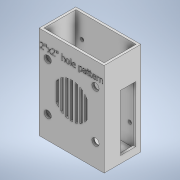
# Autodesk Inventor part: piCaseAttachesToTripodClamp
Saved by Autodesk Inventor 2022.1 (Build 261234020, 234B)
## iProperties
Created: 2021-02-07
Part Number: piCaseAttachesToTripodClamp
Material: Generic
Document SubType Name: Modeling
Designer: robst
Density: 1 g/cm^3
Appearance: Default
Author: robst
Autodesk Inventor part; units mm, degrees
ref_plane "YZ Plane" through (0, 0, 0) normal (1, 0, 0) x (0, 1, 0)
ref_plane "XZ Plane" through (0, 0, 0) normal (0, 1, 0) x (-1, 0, 0)
ref_plane "XY Plane" through (0, 0, 0) normal (0, 0, 1) x (1, 0, 0)
sketch "Sketch14" plane through (0, 0, 0) normal (0, 0, 1) x (1, 0, 0)
  line L0 (-34.54, -49.54) -> (34.54, -49.54)
  line L1 (34.54, -49.54) -> (34.54, 49.54)
  line L2 (34.54, 49.54) -> (-34.54, 49.54)
  line L3 (-34.54, 49.54) -> (-34.54, -49.54)
  line L4 (-34.54, -49.54) -> (34.54, 49.54) construction
  line L5 (34.54, -49.54) -> (-34.54, 49.54) construction
  point P0 (0, 0)
  dimension "d66" = 69.08
  dimension "d67" = 99.08
  constraints: 12 end point, 2 midpoint, 2 parallel, 1 horizontal, 1 perpendicular
  measures "d66" distance of L0.start L0.end
  measures "d67" distance of L2.end L0.start
extrude "Extrusion9" add sketch "Sketch14" against normal blind 2.54
sketch "Sketch15" plane through (0, 0, 0) normal (0, 0, 1) x (1, 0, 0)
  line L0 (-34.54, -49.54) -> (-34.54, 49.54) projected
  line L1 (34.54, 49.54) -> (34.54, -49.54) projected
  line L2 (-34.54, -49.54) -> (34.54, -49.54)
  line L3 (34.54, -49.54) -> (34.54, 49.54)
  line L4 (34.54, 49.54) -> (-34.54, 49.54)
  line L5 (-34.54, 49.54) -> (-34.54, -49.54)
  line L6 (-32, -47) -> (32, -47)
  line L7 (32, -47) -> (32, 47)
  line L8 (32, 47) -> (-32, 47)
  line L9 (-32, 47) -> (-32, -47)
  line L10 (-32, -47) -> (32, 47) construction
  line L11 (32, -47) -> (-32, 47) construction
  point P0 (0, 0)
  point P1 (34.54, -49.54)
  dimension "d70" = 64
  dimension "d71" = 94
  constraints: 20 end point, 4 parallel, 2 horizontal, 2 midpoint, 2 perpendicular
  measures "d70" distance of L6.start L6.end
  measures "d71" distance of L8.end L6.start
extrude "Extrusion10" add sketch "Sketch15" along normal blind 34
sketch "Sketch16" plane through (0, 0, 34) normal (0, 0, 1) x (1, 0, 0)
  line L0 (-34.54, -49.54) -> (-34.54, 49.54) projected
  line L1 (34.54, 49.54) -> (34.54, -49.54) projected
  line L2 (-34.54, -49.54) -> (34.54, -49.54)
  line L3 (34.54, -49.54) -> (34.54, 49.54)
  line L4 (34.54, 49.54) -> (-34.54, 49.54)
  line L5 (-34.54, 49.54) -> (-34.54, -49.54)
  point P0 (0, 0)
  point P1 (34.54, -49.54)
  constraints: 8 end point, 2 parallel, 1 horizontal, 1 perpendicular
extrude "Extrusion11" add sketch "Sketch16" along normal blind 2.54
sketch "Sketch17" plane through (-34.54, 49.54, -2.54) normal (0, 1, 0) x (1, 0, 0)
  line L0 (66.54, -2.54) -> (66.54, -36.54) projected
  line L1 (2.54, -36.54) -> (66.54, -36.54) projected
  line L2 (2.54, -2.54) -> (2.54, -36.54) projected
  line L3 (66.54, -2.54) -> (2.54, -2.54) projected
  line L4 (2.54, -36.54) -> (66.54, -36.54)
  line L5 (66.54, -36.54) -> (66.54, -2.54)
  line L6 (66.54, -2.54) -> (2.54, -2.54)
  line L7 (2.54, -2.54) -> (2.54, -36.54)
  point P0 (34.54, -2.54)
  constraints: 8 end point, 2 parallel, 1 horizontal, 1 perpendicular
extrude "Extrusion12" cut sketch "Sketch17" against normal blind 2.54
sketch "Sketch18" plane through (34.54, -49.54, -2.54) normal (1, 0, 0) x (0, 0, -1)
  line L0 (-2.54, 2.54) -> (-2.54, 99.08) projected
  line L1 (-36.54, 99.08) -> (-36.54, 2.54) projected
  line L2 (-2.54, 2.54) -> (-36.54, 2.54) projected
  line L3 (-21.54, 7.54) -> (-5.54, 7.54)
  line L4 (-5.54, 7.54) -> (-5.54, 67.54)
  line L5 (-5.54, 67.54) -> (-21.54, 67.54)
  line L6 (-21.54, 67.54) -> (-21.54, 7.54)
  line L7 (-21.54, 7.54) -> (-5.54, 67.54) construction
  line L8 (-5.54, 7.54) -> (-21.54, 67.54) construction
  line L9 (-39.08, 0) -> (-39.08, 99.08) projected
  point P0 (-2.54, 49.54)
  point P1 (-13.54, 37.54)
  dimension "d78" = 5
  dimension "d79" = 3
  dimension "d80" = 15
  dimension "d81" = 65
  constraints: 12 end point, 2 midpoint, 2 parallel, 2 perpendicular
  measures "d78" distance between parallel lines of L3 L2
  measures "d79" distance between parallel lines of L4 L0
  measures "d80" distance between parallel lines of L6 L1
  measures "d81" distance between parallel lines of L5 L2
extrude "Extrusion13" cut sketch "Sketch18" against normal blind 2.54
sketch "Sketch19" plane through (0, 0, -2.54) normal (0, 0, -1) x (-1, 0, 0)
  line L0 (-25.4, -25.4) -> (25.4, -25.4) construction
  line L1 (25.4, -25.4) -> (25.4, 25.4) construction
  line L2 (25.4, 25.4) -> (-25.4, 25.4) construction
  line L3 (-25.4, 25.4) -> (-25.4, -25.4) construction
  line L4 (-25.4, -25.4) -> (25.4, 25.4) construction
  line L5 (25.4, -25.4) -> (-25.4, 25.4) construction
  point P0 (0, 0)
  dimension "d84" = 50.8
  dimension "d85" = 50.8
  constraints: 12 end point, 2 midpoint, 2 parallel, 1 horizontal, 1 perpendicular
  measures "d84" distance of L0.start L0.end
  measures "d85" distance of L2.end L0.start
hole "Hole3" at (25.4, 25.4, -2.54) at (-25.4, 25.4, -2.54) at (-25.4, -25.4, -2.54) at (25.4, -25.4, -2.54) direction (0, 0, 1) diameter 3.81 end through all clearance for "Flat Head Machine Screw (82)" size "#6" standard "Ansi Unified Screw Threads"
sketch "Sketch22" plane through (0, 0, 36.54) normal (0, 0, 1) x (1, 0, 0)
  circle A0 centre (-25.4, 25.4) radius 1.905 projected
  circle A1 centre (25.4, 25.4) radius 1.905 projected
  circle A2 centre (25.4, -25.4) radius 1.905 projected
  circle A3 centre (-25.4, -25.4) radius 1.905 projected
  point P0 (0, 0)
  constraints: 4 coincident
hole "Hole4" at (-25.4, 25.4, 36.54) at (25.4, 25.4, 36.54) at (25.4, -25.4, 36.54) at (-25.4, -25.4, 36.54) direction (0, 0, -1) diameter 7.62 depth 2.54
sketch "Sketch23" plane through (0, 0, 36.54) normal (0, 0, 1) x (1, 0, 0)
  line L0 (-34.54, 49.54) -> (-34.54, -49.54) construction
  line L1 (-34.54, 0) -> (34.4931, 0) construction
  line L2 (32, -42) -> (32, 18) construction
  line L3 (-29.6044, 31.75) -> (-33.3638, 31.75)
  line L4 (-33.3638, 31.75) -> (-33.3638, 32.6145)
  spline S0 degree 2 poles (-33.3638, 32.6145) (-32.9587, 32.9949) (-32.2374, 33.7013) (-31.8916, 34.0817) knots 0 0 0 1 2 2 2
  spline S1 degree 2 poles (-31.8916, 34.0817) (-31.1951, 34.8474) (-30.6863, 35.7662) (-30.6863, 36.2553) knots 0 0 0 1 2 2 2
  spline S2 degree 2 poles (-30.6863, 36.2553) (-30.6863, 36.5122) (-30.8443, 36.8975) (-30.9876, 37.021) knots 0 0 0 1 2 2 2
  spline S3 degree 2 poles (-30.9876, 37.021) (-31.1309, 37.1445) (-31.5063, 37.268) (-31.7335, 37.268) knots 0 0 0 1 2 2 2
  spline S4 degree 2 poles (-31.7335, 37.268) (-31.9509, 37.268) (-32.3955, 37.1593) (-32.598, 37.0754) knots 0 0 0 1 2 2 2
  spline S5 degree 2 poles (-32.598, 37.0754) (-32.7709, 37.0062) (-33.092, 36.8086) (-33.1909, 36.7394) knots 0 0 0 1 2 2 2
  line L5 (-33.1909, 36.7394) -> (-33.2353, 36.7394)
  line L6 (-33.2353, 36.7394) -> (-33.2353, 37.6089)
  spline S6 degree 2 poles (-33.2353, 37.6089) (-32.9834, 37.7324) (-32.0793, 37.9744) (-31.6743, 37.9744) knots 0 0 0 1 2 2 2
  spline S7 degree 2 poles (-31.6743, 37.9744) (-30.8196, 37.9744) (-29.8563, 37.0704) (-29.8563, 36.2998) knots 0 0 0 1 2 2 2
  spline S8 degree 2 poles (-29.8563, 36.2998) (-29.8563, 35.9391) (-30.0243, 35.3365) (-30.1725, 35.0796) knots 0 0 0 1 2 2 2
  spline S9 degree 2 poles (-30.1725, 35.0796) (-30.3207, 34.8128) (-30.7505, 34.2892) (-30.9876, 34.0372) knots 0 0 0 1 2 2 2
  spline S10 degree 2 poles (-30.9876, 34.0372) (-31.3729, 33.6173) (-32.3165, 32.7182) (-32.598, 32.4564) knots 0 0 0 1 2 2 2
  line L7 (-32.598, 32.4564) -> (-29.6044, 32.4564)
  line L8 (-29.6044, 32.4564) -> (-29.6044, 31.75)
  line L9 (-27.8754, 38.1177) -> (-28.0532, 35.7465)
  line L10 (-28.0532, 35.7465) -> (-28.5917, 35.7465)
  line L11 (-28.5917, 35.7465) -> (-28.7695, 38.1177)
  line L12 (-28.7695, 38.1177) -> (-27.8754, 38.1177)
  line L13 (-26.3341, 38.1177) -> (-26.5119, 35.7465)
  line L14 (-26.5119, 35.7465) -> (-27.0504, 35.7465)
  line L15 (-27.0504, 35.7465) -> (-27.2282, 38.1177)
  line L16 (-27.2282, 38.1177) -> (-26.3341, 38.1177)
  line L17 (-21.7596, 31.75) -> (-22.7032, 31.75)
  line L18 (-22.7032, 31.75) -> (-23.8147, 33.4691)
  line L19 (-23.8147, 33.4691) -> (-24.9558, 31.75)
  line L20 (-24.9558, 31.75) -> (-25.8302, 31.75)
  line L21 (-25.8302, 31.75) -> (-24.2445, 34.0175)
  line L22 (-24.2445, 34.0175) -> (-25.8154, 36.3245)
  line L23 (-25.8154, 36.3245) -> (-24.8718, 36.3245)
  line L24 (-24.8718, 36.3245) -> (-23.7653, 34.6202)
  line L25 (-23.7653, 34.6202) -> (-22.634, 36.3245)
  line L26 (-22.634, 36.3245) -> (-21.7596, 36.3245)
  line L27 (-21.7596, 36.3245) -> (-23.3355, 34.0669)
  line L28 (-23.3355, 34.0669) -> (-21.7596, 31.75)
  line L29 (-17.5161, 31.75) -> (-21.2755, 31.75)
  line L30 (-21.2755, 31.75) -> (-21.2755, 32.6145)
  spline S11 degree 2 poles (-21.2755, 32.6145) (-20.8704, 32.9949) (-20.1492, 33.7013) (-19.8034, 34.0817) knots 0 0 0 1 2 2 2
  spline S12 degree 2 poles (-19.8034, 34.0817) (-19.1068, 34.8474) (-18.598, 35.7662) (-18.598, 36.2553) knots 0 0 0 1 2 2 2
  spline S13 degree 2 poles (-18.598, 36.2553) (-18.598, 36.5122) (-18.7561, 36.8975) (-18.8993, 37.021) knots 0 0 0 1 2 2 2
  spline S14 degree 2 poles (-18.8993, 37.021) (-19.0426, 37.1445) (-19.418, 37.268) (-19.6453, 37.268) knots 0 0 0 1 2 2 2
  spline S15 degree 2 poles (-19.6453, 37.268) (-19.8626, 37.268) (-20.3072, 37.1593) (-20.5098, 37.0754) knots 0 0 0 1 2 2 2
  spline S16 degree 2 poles (-20.5098, 37.0754) (-20.6827, 37.0062) (-21.0038, 36.8086) (-21.1026, 36.7394) knots 0 0 0 1 2 2 2
  line L31 (-21.1026, 36.7394) -> (-21.1471, 36.7394)
  line L32 (-21.1471, 36.7394) -> (-21.1471, 37.6089)
  spline S17 degree 2 poles (-21.1471, 37.6089) (-20.8951, 37.7324) (-19.9911, 37.9744) (-19.586, 37.9744) knots 0 0 0 1 2 2 2
  spline S18 degree 2 poles (-19.586, 37.9744) (-18.7314, 37.9744) (-17.7681, 37.0704) (-17.7681, 36.2998) knots 0 0 0 1 2 2 2
  spline S19 degree 2 poles (-17.7681, 36.2998) (-17.7681, 35.9391) (-17.936, 35.3365) (-18.0842, 35.0796) knots 0 0 0 1 2 2 2
  spline S20 degree 2 poles (-18.0842, 35.0796) (-18.2324, 34.8128) (-18.6622, 34.2892) (-18.8993, 34.0372) knots 0 0 0 1 2 2 2
  spline S21 degree 2 poles (-18.8993, 34.0372) (-19.2847, 33.6173) (-20.2282, 32.7182) (-20.5098, 32.4564) knots 0 0 0 1 2 2 2
  line L33 (-20.5098, 32.4564) -> (-17.5161, 32.4564)
  line L34 (-17.5161, 32.4564) -> (-17.5161, 31.75)
  line L35 (-14.2458, 38.1177) -> (-14.4237, 35.7465)
  line L36 (-14.4237, 35.7465) -> (-14.9621, 35.7465)
  line L37 (-14.9621, 35.7465) -> (-15.14, 38.1177)
  line L38 (-15.14, 38.1177) -> (-14.2458, 38.1177)
  line L39 (-15.7871, 38.1177) -> (-15.965, 35.7465)
  line L40 (-15.965, 35.7465) -> (-16.5034, 35.7465)
  line L41 (-16.5034, 35.7465) -> (-16.6813, 38.1177)
  line L42 (-16.6813, 38.1177) -> (-15.7871, 38.1177)
  line L43 (-7.0136, 31.75) -> (-7.7843, 31.75)
  line L44 (-7.7843, 31.75) -> (-7.7843, 34.3583)
  spline S22 degree 2 poles (-7.7843, 34.3583) (-7.7843, 34.6745) (-7.8435, 35.2179) (-7.9325, 35.3809) knots 0 0 0 1 2 2 2
  spline S23 degree 2 poles (-7.9325, 35.3809) (-8.0263, 35.5538) (-8.3622, 35.7218) (-8.6488, 35.7218) knots 0 0 0 1 2 2 2
  spline S24 degree 2 poles (-8.6488, 35.7218) (-8.9353, 35.7218) (-9.5429, 35.4155) (-9.8344, 35.1685) knots 0 0 0 1 2 2 2
  line L45 (-9.8344, 35.1685) -> (-9.8344, 31.75)
  line L46 (-9.8344, 31.75) -> (-10.605, 31.75)
  line L47 (-10.605, 31.75) -> (-10.605, 38.1177)
  line L48 (-10.605, 38.1177) -> (-9.8344, 38.1177)
  line L49 (-9.8344, 38.1177) -> (-9.8344, 35.8156)
  spline S25 degree 2 poles (-9.8344, 35.8156) (-9.4886, 36.1269) (-8.8217, 36.4529) (-8.4462, 36.4529) knots 0 0 0 1 2 2 2
  spline S26 degree 2 poles (-8.4462, 36.4529) (-7.7744, 36.4529) (-7.0136, 35.5637) (-7.0136, 34.719) knots 0 0 0 1 2 2 2
  line L50 (-7.0136, 34.719) -> (-7.0136, 31.75)
  spline S27 degree 2 poles (-2.1724, 34.0372) (-2.1724, 32.8813) (-3.2839, 31.6216) (-4.2126, 31.6216) knots 0 0 0 1 2 2 2
  spline S28 degree 2 poles (-4.2126, 31.6216) (-5.166, 31.6216) (-6.2578, 32.9208) (-6.2578, 34.0372) knots 0 0 0 1 2 2 2
  spline S29 degree 2 poles (-6.2578, 34.0372) (-6.2578, 35.1833) (-5.1315, 36.4529) (-4.2126, 36.4529) knots 0 0 0 1 2 2 2
  spline S30 degree 2 poles (-4.2126, 36.4529) (-3.2839, 36.4529) (-2.1724, 35.1883) (-2.1724, 34.0372) knots 0 0 0 1 2 2 2
  spline S31 degree 2 poles (-2.9677, 34.0372) (-2.9677, 34.9264) (-3.6149, 35.7909) (-4.2126, 35.7909) knots 0 0 0 1 2 2 2
  spline S32 degree 2 poles (-4.2126, 35.7909) (-4.8104, 35.7909) (-5.4624, 34.9264) (-5.4624, 34.0372) knots 0 0 0 1 2 2 2
  spline S33 degree 2 poles (-5.4624, 34.0372) (-5.4624, 33.1727) (-4.8104, 32.2835) (-4.2126, 32.2835) knots 0 0 0 1 2 2 2
  spline S34 degree 2 poles (-4.2126, 32.2835) (-3.6198, 32.2835) (-2.9677, 33.1579) (-2.9677, 34.0372) knots 0 0 0 1 2 2 2
  line L51 (-0.5965, 31.75) -> (-1.3672, 31.75)
  line L52 (-1.3672, 31.75) -> (-1.3672, 38.1177)
  line L53 (-1.3672, 38.1177) -> (-0.5965, 38.1177)
  line L54 (-0.5965, 38.1177) -> (-0.5965, 31.75)
  spline S35 degree 2 poles (2.5206, 31.6463) (1.424, 31.6463) (0.2186, 32.8763) (0.2186, 34.0125) knots 0 0 0 1 2 2 2
  spline S36 degree 2 poles (0.2186, 34.0125) (0.2186, 35.129) (1.3894, 36.4529) (2.3329, 36.4529) knots 0 0 0 1 2 2 2
  spline S37 degree 2 poles (2.3329, 36.4529) (2.7578, 36.4529) (3.4148, 36.2059) (3.6569, 35.9441) knots 0 0 0 1 2 2 2
  spline S38 degree 2 poles (3.6569, 35.9441) (3.9039, 35.6823) (4.1657, 34.9264) (4.1657, 34.3781) knots 0 0 0 1 2 2 2
  line L55 (4.1657, 34.3781) -> (4.1657, 33.9582)
  line L56 (4.1657, 33.9582) -> (0.9991, 33.9582)
  spline S39 degree 2 poles (0.9991, 33.9582) (0.9991, 33.1628) (1.7994, 32.3181) (2.5108, 32.3181) knots 0 0 0 1 2 2 2
  spline S40 degree 2 poles (2.5108, 32.3181) (2.7627, 32.3181) (3.2518, 32.4317) (3.4494, 32.5206) knots 0 0 0 1 2 2 2
  spline S41 degree 2 poles (3.4494, 32.5206) (3.6569, 32.6194) (3.9434, 32.7923) (4.0372, 32.8714) knots 0 0 0 1 2 2 2
  line L57 (4.0372, 32.8714) -> (4.0817, 32.8714)
  line L58 (4.0817, 32.8714) -> (4.0817, 32.0316)
  spline S42 degree 2 poles (4.0817, 32.0316) (3.9483, 31.9772) (3.5432, 31.8192) (3.3851, 31.7747) knots 0 0 0 1 2 2 2
  spline S43 degree 2 poles (3.3851, 31.7747) (3.1628, 31.7105) (2.7973, 31.6463) (2.5206, 31.6463) knots 0 0 0 1 2 2 2
  spline S44 degree 2 poles (3.4148, 34.5461) (3.4049, 34.8573) (3.2765, 35.3118) (3.153, 35.4649) knots 0 0 0 1 2 2 2
  spline S45 degree 2 poles (3.153, 35.4649) (3.0196, 35.6378) (2.5997, 35.8206) (2.2885, 35.8206) knots 0 0 0 1 2 2 2
  spline S46 degree 2 poles (2.2885, 35.8206) (1.9822, 35.8206) (1.5524, 35.6378) (1.3746, 35.46) knots 0 0 0 1 2 2 2
  spline S47 degree 2 poles (1.3746, 35.46) (1.2017, 35.2772) (1.0238, 34.8375) (0.9991, 34.5461) knots 0 0 0 1 2 2 2
  line L59 (0.9991, 34.5461) -> (3.4148, 34.5461)
  spline S48 degree 2 poles (11.3979, 34.1607) (11.3979, 33.0146) (10.3061, 31.6611) (9.4713, 31.6611) knots 0 0 0 1 2 2 2
  spline S49 degree 2 poles (9.4713, 31.6611) (9.1304, 31.6611) (8.6068, 31.8192) (8.3351, 31.9822) knots 0 0 0 1 2 2 2
  line L60 (8.3351, 31.9822) -> (8.3351, 30.0654)
  line L61 (8.3351, 30.0654) -> (7.5644, 30.0654)
  line L62 (7.5644, 30.0654) -> (7.5644, 36.3245)
  line L63 (7.5644, 36.3245) -> (8.3351, 36.3245)
  line L64 (8.3351, 36.3245) -> (8.3351, 35.8453)
  spline S50 degree 2 poles (8.3351, 35.8453) (8.6216, 36.1071) (9.3231, 36.4529) (9.7331, 36.4529) knots 0 0 0 1 2 2 2
  spline S51 degree 2 poles (9.7331, 36.4529) (10.5186, 36.4529) (11.3979, 35.208) (11.3979, 34.1607) knots 0 0 0 1 2 2 2
  spline S52 degree 2 poles (10.6025, 34.0718) (10.6025, 34.8573) (10.1036, 35.7218) (9.5454, 35.7218) knots 0 0 0 1 2 2 2
  spline S53 degree 2 poles (9.5454, 35.7218) (9.2193, 35.7218) (8.6068, 35.4303) (8.3351, 35.2031) knots 0 0 0 1 2 2 2
  line L65 (8.3351, 35.2031) -> (8.3351, 32.6046)
  spline S54 degree 2 poles (8.3351, 32.6046) (8.6364, 32.4614) (9.0662, 32.3527) (9.3428, 32.3527) knots 0 0 0 1 2 2 2
  spline S55 degree 2 poles (9.3428, 32.3527) (9.9406, 32.3527) (10.6025, 33.232) (10.6025, 34.0718) knots 0 0 0 1 2 2 2
  spline S56 degree 2 poles (14.7472, 32.2341) (14.6534, 32.165) (14.3372, 31.918) (14.189, 31.8439) knots 0 0 0 1 2 2 2
  spline S57 degree 2 poles (14.189, 31.8439) (13.9865, 31.7352) (13.6061, 31.6216) (13.2603, 31.6216) knots 0 0 0 1 2 2 2
  spline S58 degree 2 poles (13.2603, 31.6216) (12.9787, 31.6216) (12.4699, 31.834) (12.2772, 32.0266) knots 0 0 0 1 2 2 2
  spline S59 degree 2 poles (12.2772, 32.0266) (12.0944, 32.2144) (11.8721, 32.7676) (11.8721, 33.0739) knots 0 0 0 1 2 2 2
  spline S60 degree 2 poles (11.8721, 33.0739) (11.8721, 33.5482) (12.2723, 34.22) (12.707, 34.4127) knots 0 0 0 1 2 2 2
  spline S61 degree 2 poles (12.707, 34.4127) (13.0923, 34.5905) (14.1396, 34.7239) (14.7472, 34.7585) knots 0 0 0 1 2 2 2
  line L66 (14.7472, 34.7585) -> (14.7472, 34.9067)
  spline S62 degree 2 poles (14.7472, 34.9067) (14.7472, 35.1734) (14.5842, 35.5044) (14.436, 35.5983) knots 0 0 0 1 2 2 2
  spline S63 degree 2 poles (14.436, 35.5983) (14.2878, 35.6921) (13.863, 35.7514) (13.6357, 35.7514) knots 0 0 0 1 2 2 2
  spline S64 degree 2 poles (13.6357, 35.7514) (13.369, 35.7514) (12.6477, 35.5933) (12.2871, 35.4402) knots 0 0 0 1 2 2 2
  line L67 (12.2871, 35.4402) -> (12.2426, 35.4402)
  line L68 (12.2426, 35.4402) -> (12.2426, 36.2257)
  spline S65 degree 2 poles (12.2426, 36.2257) (12.455, 36.2849) (13.2504, 36.4332) (13.6407, 36.4332) knots 0 0 0 1 2 2 2
  spline S66 degree 2 poles (13.6407, 36.4332) (14.1149, 36.4332) (14.762, 36.2849) (15.0189, 36.0923) knots 0 0 0 1 2 2 2
  spline S67 degree 2 poles (15.0189, 36.0923) (15.2709, 35.9046) (15.5179, 35.3068) (15.5179, 34.877) knots 0 0 0 1 2 2 2
  line L69 (15.5179, 34.877) -> (15.5179, 31.75)
  line L70 (15.5179, 31.75) -> (14.7472, 31.75)
  line L71 (14.7472, 31.75) -> (14.7472, 32.2341)
  line L72 (14.7472, 32.8763) -> (14.7472, 34.1459)
  spline S68 degree 2 poles (14.7472, 34.1459) (14.4706, 34.1212) (13.6357, 34.0372) (13.3739, 33.9582) knots 0 0 0 1 2 2 2
  spline S69 degree 2 poles (13.3739, 33.9582) (13.0676, 33.8643) (12.6675, 33.4741) (12.6675, 33.1283) knots 0 0 0 1 2 2 2
  spline S70 degree 2 poles (12.6675, 33.1283) (12.6675, 32.7331) (13.1121, 32.3329) (13.5369, 32.3329) knots 0 0 0 1 2 2 2
  spline S71 degree 2 poles (13.5369, 32.3329) (13.8975, 32.3329) (14.4903, 32.6441) (14.7472, 32.8763) knots 0 0 0 1 2 2 2
  spline S72 degree 2 poles (17.9829, 31.6611) (17.3556, 31.6611) (16.6491, 32.3774) (16.6491, 33.153) knots 0 0 0 1 2 2 2
  line L73 (16.6491, 33.153) -> (16.6491, 35.6872)
  line L74 (16.6491, 35.6872) -> (16.1304, 35.6872)
  line L75 (16.1304, 35.6872) -> (16.1304, 36.3245)
  line L76 (16.1304, 36.3245) -> (16.6491, 36.3245)
  line L77 (16.6491, 36.3245) -> (16.6491, 37.6385)
  line L78 (16.6491, 37.6385) -> (17.4198, 37.6385)
  line L79 (17.4198, 37.6385) -> (17.4198, 36.3245)
  line L80 (17.4198, 36.3245) -> (18.8376, 36.3245)
  line L81 (18.8376, 36.3245) -> (18.8376, 35.6872)
  line L82 (18.8376, 35.6872) -> (17.4198, 35.6872)
  line L83 (17.4198, 35.6872) -> (17.4198, 33.5087)
  spline S73 degree 2 poles (17.4198, 33.5087) (17.4198, 33.1628) (17.4445, 32.7825) (17.5285, 32.6194) knots 0 0 0 1 2 2 2
  spline S74 degree 2 poles (17.5285, 32.6194) (17.5976, 32.4762) (17.9088, 32.3329) (18.1756, 32.3329) knots 0 0 0 1 2 2 2
  spline S75 degree 2 poles (18.1756, 32.3329) (18.3633, 32.3329) (18.7141, 32.4465) (18.7931, 32.4811) knots 0 0 0 1 2 2 2
  line L84 (18.7931, 32.4811) -> (18.8376, 32.4811)
  line L85 (18.8376, 32.4811) -> (18.8376, 31.7895)
  spline S76 degree 2 poles (18.8376, 31.7895) (18.6202, 31.7302) (18.1756, 31.6611) (17.9829, 31.6611) knots 0 0 0 1 2 2 2
  spline S77 degree 2 poles (20.7889, 31.6611) (20.1615, 31.6611) (19.4551, 32.3774) (19.4551, 33.153) knots 0 0 0 1 2 2 2
  line L86 (19.4551, 33.153) -> (19.4551, 35.6872)
  line L87 (19.4551, 35.6872) -> (18.9364, 35.6872)
  line L88 (18.9364, 35.6872) -> (18.9364, 36.3245)
  line L89 (18.9364, 36.3245) -> (19.4551, 36.3245)
  line L90 (19.4551, 36.3245) -> (19.4551, 37.6385)
  line L91 (19.4551, 37.6385) -> (20.2257, 37.6385)
  line L92 (20.2257, 37.6385) -> (20.2257, 36.3245)
  line L93 (20.2257, 36.3245) -> (21.6435, 36.3245)
  line L94 (21.6435, 36.3245) -> (21.6435, 35.6872)
  line L95 (21.6435, 35.6872) -> (20.2257, 35.6872)
  line L96 (20.2257, 35.6872) -> (20.2257, 33.5087)
  spline S78 degree 2 poles (20.2257, 33.5087) (20.2257, 33.1628) (20.2504, 32.7825) (20.3344, 32.6194) knots 0 0 0 1 2 2 2
  spline S79 degree 2 poles (20.3344, 32.6194) (20.4036, 32.4762) (20.7148, 32.3329) (20.9815, 32.3329) knots 0 0 0 1 2 2 2
  spline S80 degree 2 poles (20.9815, 32.3329) (21.1693, 32.3329) (21.52, 32.4465) (21.599, 32.4811) knots 0 0 0 1 2 2 2
  line L97 (21.599, 32.4811) -> (21.6435, 32.4811)
  line L98 (21.6435, 32.4811) -> (21.6435, 31.7895)
  spline S81 degree 2 poles (21.6435, 31.7895) (21.4261, 31.7302) (20.9815, 31.6611) (20.7889, 31.6611) knots 0 0 0 1 2 2 2
  spline S82 degree 2 poles (24.1975, 31.6463) (23.1008, 31.6463) (21.8955, 32.8763) (21.8955, 34.0125) knots 0 0 0 1 2 2 2
  spline S83 degree 2 poles (21.8955, 34.0125) (21.8955, 35.129) (23.0662, 36.4529) (24.0098, 36.4529) knots 0 0 0 1 2 2 2
  spline S84 degree 2 poles (24.0098, 36.4529) (24.4346, 36.4529) (25.0917, 36.2059) (25.3337, 35.9441) knots 0 0 0 1 2 2 2
  spline S85 degree 2 poles (25.3337, 35.9441) (25.5807, 35.6823) (25.8425, 34.9264) (25.8425, 34.3781) knots 0 0 0 1 2 2 2
  line L99 (25.8425, 34.3781) -> (25.8425, 33.9582)
  line L100 (25.8425, 33.9582) -> (22.676, 33.9582)
  spline S86 degree 2 poles (22.676, 33.9582) (22.676, 33.1628) (23.4763, 32.3181) (24.1876, 32.3181) knots 0 0 0 1 2 2 2
  spline S87 degree 2 poles (24.1876, 32.3181) (24.4396, 32.3181) (24.9286, 32.4317) (25.1262, 32.5206) knots 0 0 0 1 2 2 2
  spline S88 degree 2 poles (25.1262, 32.5206) (25.3337, 32.6194) (25.6202, 32.7923) (25.7141, 32.8714) knots 0 0 0 1 2 2 2
  line L101 (25.7141, 32.8714) -> (25.7586, 32.8714)
  line L102 (25.7586, 32.8714) -> (25.7586, 32.0316)
  spline S89 degree 2 poles (25.7586, 32.0316) (25.6252, 31.9772) (25.2201, 31.8192) (25.062, 31.7747) knots 0 0 0 1 2 2 2
  spline S90 degree 2 poles (25.062, 31.7747) (24.8397, 31.7105) (24.4741, 31.6463) (24.1975, 31.6463) knots 0 0 0 1 2 2 2
  spline S91 degree 2 poles (25.0917, 34.5461) (25.0818, 34.8573) (24.9533, 35.3118) (24.8298, 35.4649) knots 0 0 0 1 2 2 2
  spline S92 degree 2 poles (24.8298, 35.4649) (24.6964, 35.6378) (24.2765, 35.8206) (23.9653, 35.8206) knots 0 0 0 1 2 2 2
  spline S93 degree 2 poles (23.9653, 35.8206) (23.659, 35.8206) (23.2293, 35.6378) (23.0514, 35.46) knots 0 0 0 1 2 2 2
  spline S94 degree 2 poles (23.0514, 35.46) (22.8785, 35.2772) (22.7007, 34.8375) (22.676, 34.5461) knots 0 0 0 1 2 2 2
  line L103 (22.676, 34.5461) -> (25.0917, 34.5461)
  line L104 (29.0486, 35.4995) -> (29.0091, 35.4995)
  spline S95 degree 2 poles (29.0091, 35.4995) (28.9202, 35.5242) (28.7275, 35.5341) (28.5941, 35.5341) knots 0 0 0 1 2 2 2
  spline S96 degree 2 poles (28.5941, 35.5341) (28.2829, 35.5341) (27.6703, 35.2624) (27.3937, 34.9956) knots 0 0 0 1 2 2 2
  line L105 (27.3937, 34.9956) -> (27.3937, 31.75)
  line L106 (27.3937, 31.75) -> (26.6231, 31.75)
  line L107 (26.6231, 31.75) -> (26.6231, 36.3245)
  line L108 (26.6231, 36.3245) -> (27.3937, 36.3245)
  line L109 (27.3937, 36.3245) -> (27.3937, 35.6427)
  spline S97 degree 2 poles (27.3937, 35.6427) (27.8136, 36.0182) (28.441, 36.3245) (28.7374, 36.3245) knots 0 0 0 1 2 2 2
  spline S98 degree 2 poles (28.7374, 36.3245) (28.856, 36.3245) (28.9745, 36.3146) (29.0486, 36.2998) knots 0 0 0 1 2 2 2
  line L110 (29.0486, 36.2998) -> (29.0486, 35.4995)
  line L111 (33.2378, 31.75) -> (32.4671, 31.75)
  line L112 (32.4671, 31.75) -> (32.4671, 34.3583)
  spline S99 degree 2 poles (32.4671, 34.3583) (32.4671, 34.6745) (32.4078, 35.2179) (32.3189, 35.3809) knots 0 0 0 1 2 2 2
  spline S100 degree 2 poles (32.3189, 35.3809) (32.2251, 35.5538) (31.8891, 35.7218) (31.6026, 35.7218) knots 0 0 0 1 2 2 2
  spline S101 degree 2 poles (31.6026, 35.7218) (31.3161, 35.7218) (30.7085, 35.4155) (30.417, 35.1685) knots 0 0 0 1 2 2 2
  line L113 (30.417, 35.1685) -> (30.417, 31.75)
  line L114 (30.417, 31.75) -> (29.6464, 31.75)
  line L115 (29.6464, 31.75) -> (29.6464, 36.3245)
  line L116 (29.6464, 36.3245) -> (30.417, 36.3245)
  line L117 (30.417, 36.3245) -> (30.417, 35.8156)
  spline S102 degree 2 poles (30.417, 35.8156) (30.7628, 36.1269) (31.4297, 36.4529) (31.8052, 36.4529) knots 0 0 0 1 2 2 2
  spline S103 degree 2 poles (31.8052, 36.4529) (32.477, 36.4529) (33.2378, 35.5637) (33.2378, 34.719) knots 0 0 0 1 2 2 2
  line L118 (33.2378, 34.719) -> (33.2378, 31.75)
  point P0 (0, 0)
  constraints: 2 end point, 1 horizontal, 1 midpoint, 1 perpendicular
extrude "Extrusion14" cut sketch "Sketch23" against normal blind 1.27
sketch "Sketch24" plane through (0, 0, 36.54) normal (0, 0, 1) x (1, 0, 0)
  line L0 (-1.27, 19.0076) -> (-1.27, -19.0076)
  line L1 (0, 0) -> (0, 19.05) construction
  line L2 (-3.81, 18.6651) -> (-3.81, -18.6651)
  line L3 (-6.35, 17.9605) -> (-6.35, -17.9605)
  line L4 (-8.89, -16.8485) -> (-8.89, 16.8485)
  line L5 (-11.43, 15.24) -> (-11.43, -15.24)
  line L6 (-13.97, -12.9515) -> (-13.97, 12.9515)
  line L7 (-16.51, -9.5038) -> (-16.51, 9.5038)
  arc A0 (-6.35, -17.9605) -> (-3.81, -18.6651) centre (0, 0) ccw
  arc A1 (-11.43, -15.24) -> (-8.89, -16.8485) centre (0, 0) ccw
  arc A2 (-16.51, -9.5038) -> (-13.97, -12.9515) centre (0, 0) ccw
  arc A3 (-13.97, 12.9515) -> (-16.51, 9.5038) centre (0, 0) ccw
  arc A4 (-3.81, 18.6651) -> (-6.35, 17.9605) centre (0, 0) ccw
  arc A5 (-8.89, 16.8485) -> (-11.43, 15.24) centre (0, 0) ccw
  arc A6 (-1.27, -19.0076) -> (0, -19.05) centre (0, 0) ccw
  arc A7 (0, 19.05) -> (-1.27, 19.0076) centre (0, 0) ccw
  line L8 (0, -19.05) -> (0, 19.05)
  dimension "d104" = 2.54
  dimension "d105" = 2.54
  dimension "d106" = 2.54
  dimension "d107" = 2.54
  dimension "d108" = 2.54
  dimension "d109" = 2.54
  constraints: 18 end point, 16 point on circle, 8 centre point, 8 vertical, 1 coincident, 1 collinear
  measures "d104" distance between parallel lines of L2 L0
  measures "d105" distance between parallel lines of L3 L2
  measures "d106" distance between parallel lines of L4 L3
  measures "d107" distance between parallel lines of L5 L4
  measures "d108" distance between parallel lines of L6 L5
  measures "d109" distance between parallel lines of L7 L6
extrude "Extrusion15" cut sketch "Sketch24" against normal up to next
mirror "Mirror2" about plane through (0, 19.05, 36.54) normal (-1, 0, 0) of "Extrusion15"
equation "\"d66\" = piBoxExteriorWidth"
equation "\"d67\" = piBoxExteriorLength"
equation "\"d68\" = piBoxWallThickness"
equation "\"d70\" = piBoxInteriorWidth"
equation "\"d71\" = piBoxInteriorLength"
equation "\"d72\" = piBoxInteriorHeight"
equation "\"d74\" = piBoxWallThickness"
equation "\"d76\" = piBoxWallThickness"
equation "\"d82\" = piBoxWallThickness"
equation "\"piBoxInteriorLength\" = 94"
equation "\"piBoxInteriorWidth\" = 64"
equation "\"piBoxInteriorHeight\" = 34"
equation "\"piBoxThickness\" = 3.175"
equation "\"piBoxWallThickness\" = 2.54"
equation "\"piBoxExteriorLength\" = piBoxInteriorLength + 2 * piBoxWallThickness"
equation "\"piBoxExteriorHeight\" = piBoxInteriorHeight + piBoxWallThickness"
equation "\"piBoxExteriorWidth\" = piBoxInteriorWidth + 2 * piBoxWallThickness"
body "Solid1"
body "Solid2"
